Autodesk Fusion 360 part; units mm, degrees
(part 2 of 10)
  line L884 (3.8217, -13.8798) -> (4.0299, -13.8798)
  line L885 (4.0299, -13.8798) -> (4.0984, -13.8456)
  line L886 (4.0984, -13.8456) -> (4.1288, -13.8152)
  line L887 (4.1288, -13.8152) -> (4.1631, -13.7466)
  line L888 (4.1631, -13.7466) -> (4.1631, -13.6868)
  line L889 (4.1631, -13.6868) -> (4.1288, -13.6183)
  line L890 (4.1288, -13.6183) -> (4.0984, -13.5879)
  line L891 (4.0984, -13.5879) -> (4.0214, -13.5494)
  line L892 (4.0214, -13.5494) -> (3.839, -13.5038)
  line L893 (3.839, -13.5038) -> (3.8379, -13.5034)
  line L894 (3.8379, -13.5034) -> (3.8373, -13.5033)
  line L895 (3.8373, -13.5033) -> (3.8312, -13.501)
  line L896 (3.8312, -13.501) -> (3.8251, -13.4988)
  line L897 (3.8251, -13.4988) -> (3.8247, -13.4985)
  line L898 (3.8247, -13.4985) -> (3.8236, -13.4981)
  line L899 (3.8236, -13.4981) -> (3.7284, -13.4505)
  line L900 (3.7284, -13.4505) -> (3.7221, -13.4465)
  line L901 (3.7221, -13.4465) -> (3.7202, -13.4458)
  line L902 (3.7202, -13.4458) -> (3.7182, -13.4441)
  line L903 (3.7182, -13.4441) -> (3.7159, -13.4426)
  line L904 (3.7159, -13.4426) -> (3.7146, -13.4411)
  line L905 (3.7146, -13.4411) -> (3.7089, -13.4364)
  line L906 (3.7089, -13.4364) -> (3.6613, -13.3888)
  line L907 (3.6613, -13.3888) -> (3.6565, -13.3831)
  line L908 (3.6565, -13.3831) -> (3.655, -13.3818)
  line L909 (3.655, -13.3818) -> (3.6536, -13.3795)
  line L910 (3.6536, -13.3795) -> (3.6519, -13.3774)
  line L911 (3.6519, -13.3774) -> (3.6512, -13.3756)
  line L912 (3.6512, -13.3756) -> (3.6472, -13.3693)
  line L913 (3.6472, -13.3693) -> (3.5996, -13.2741)
  line L914 (3.5996, -13.2741) -> (3.5943, -13.2603)
  line L915 (3.5943, -13.2603) -> (3.5941, -13.2577)
  line L916 (3.5941, -13.2577) -> (3.5931, -13.2552)
  line L917 (3.5931, -13.2552) -> (3.5917, -13.2405)
  line L918 (3.5917, -13.2405) -> (3.5917, -13.1453)
  line L919 (3.5917, -13.1453) -> (3.5931, -13.1307)
  line L920 (3.5931, -13.1307) -> (3.5941, -13.1282)
  line L921 (3.5941, -13.1282) -> (3.5943, -13.1255)
  line L922 (3.5943, -13.1255) -> (3.5996, -13.1118)
  line L923 (3.5996, -13.1118) -> (3.6472, -13.0165)
  line L924 (3.6472, -13.0165) -> (3.6512, -13.0102)
  line L925 (3.6512, -13.0102) -> (3.6519, -13.0084)
  line L926 (3.6519, -13.0084) -> (3.6536, -13.0063)
  line L927 (3.6536, -13.0063) -> (3.655, -13.0041)
  line L928 (3.655, -13.0041) -> (3.6565, -13.0028)
  line L929 (3.6565, -13.0028) -> (3.6613, -12.997)
  line L930 (3.6613, -12.997) -> (3.7089, -12.9494)
  line L931 (3.7089, -12.9494) -> (3.7146, -12.9447)
  line L932 (3.7146, -12.9447) -> (3.7159, -12.9432)
  line L933 (3.7159, -12.9432) -> (3.7182, -12.9418)
  line L934 (3.7182, -12.9418) -> (3.7202, -12.9401)
  line L935 (3.7202, -12.9401) -> (3.7221, -12.9393)
  line L936 (3.7221, -12.9393) -> (3.7284, -12.9354)
  line L937 (3.7284, -12.9354) -> (3.8236, -12.8877)
  line L938 (3.8236, -12.8877) -> (3.8373, -12.8825)
  line L939 (3.8373, -12.8825) -> (3.84, -12.8823)
  line L940 (3.84, -12.8823) -> (3.8425, -12.8813)
  line L941 (3.8425, -12.8813) -> (3.8571, -12.8798)
  line L942 (3.8571, -12.8798) -> (4.0952, -12.8798)
  line L943 (4.0952, -12.8798) -> (4.1026, -12.8805)
  line L944 (5.4598, -12.8867) -> (5.4836, -12.9038)
  line L945 (5.4836, -12.9038) -> (5.4989, -12.9287)
  line L946 (5.4989, -12.9287) -> (5.5035, -12.9576)
  line L947 (5.5035, -12.9576) -> (5.5015, -12.9722)
  line L948 (5.5015, -12.9722) -> (5.2634, -13.9722)
  line L949 (5.2634, -13.9722) -> (5.2617, -13.9772)
  line L950 (5.2617, -13.9772) -> (5.2615, -13.979)
  line L951 (5.2615, -13.979) -> (5.2605, -13.9806)
  line L952 (5.2605, -13.9806) -> (5.2586, -13.9861)
  line L953 (5.2586, -13.9861) -> (5.2523, -13.9949)
  line L954 (5.2523, -13.9949) -> (5.2468, -14.0043)
  line L955 (5.2468, -14.0043) -> (5.2437, -14.0067)
  line L956 (5.2437, -14.0067) -> (5.2415, -14.0098)
  line L957 (5.2415, -14.0098) -> (5.2322, -14.0155)
  line L958 (5.2322, -14.0155) -> (5.2236, -14.0221)
  line L959 (5.2236, -14.0221) -> (5.2198, -14.0231)
  line L960 (5.2198, -14.0231) -> (5.2166, -14.0251)
  line L961 (5.2166, -14.0251) -> (5.2058, -14.0269)
  line L962 (5.2058, -14.0269) -> (5.1953, -14.0297)
  line L963 (5.1953, -14.0297) -> (5.1915, -14.0292)
  line L964 (5.1915, -14.0292) -> (5.1877, -14.0298)
  line L965 (5.1877, -14.0298) -> (5.1771, -14.0272)
  line L966 (5.1771, -14.0272) -> (5.1663, -14.0258)
  line L967 (5.1663, -14.0258) -> (5.163, -14.0239)
  line L968 (5.163, -14.0239) -> (5.1592, -14.023)
  line L969 (5.1592, -14.023) -> (5.1504, -14.0166)
  line L970 (5.1504, -14.0166) -> (5.141, -14.0111)
  line L971 (5.141, -14.0111) -> (5.1386, -14.0081)
  line L972 (5.1386, -14.0081) -> (5.1355, -14.0058)
  line L973 (5.1355, -14.0058) -> (5.1298, -13.9966)
  line L974 (5.1298, -13.9966) -> (5.1232, -13.9879)
  line L975 (5.1232, -13.9879) -> (5.1211, -13.9825)
  line L976 (5.1211, -13.9825) -> (5.1202, -13.9809)
  line L977 (5.1202, -13.9809) -> (5.1199, -13.9791)
  line L978 (5.1199, -13.9791) -> (5.118, -13.9741)
  line L979 (5.118, -13.9741) -> (5, -13.5316)
  line L980 (5, -13.5316) -> (4.882, -13.9741)
  line L981 (4.882, -13.9741) -> (4.8801, -13.9791)
  line L982 (4.8801, -13.9791) -> (4.8798, -13.9809)
  line L983 (4.8798, -13.9809) -> (4.8789, -13.9825)
  line L984 (4.8789, -13.9825) -> (4.8768, -13.9879)
  line L985 (4.8768, -13.9879) -> (4.8702, -13.9966)
  line L986 (4.8702, -13.9966) -> (4.8645, -14.0058)
  line L987 (4.8645, -14.0058) -> (4.8614, -14.0081)
  line L988 (4.8614, -14.0081) -> (4.859, -14.0111)
  line L989 (4.859, -14.0111) -> (4.8496, -14.0166)
  line L990 (4.8496, -14.0166) -> (4.8408, -14.023)
  line L991 (4.8408, -14.023) -> (4.837, -14.0239)
  line L992 (4.837, -14.0239) -> (4.8337, -14.0258)
  line L993 (4.8337, -14.0258) -> (4.8229, -14.0272)
  line L994 (4.8229, -14.0272) -> (4.8123, -14.0298)
  line L995 (4.8123, -14.0298) -> (4.8085, -14.0292)
  line L996 (4.8085, -14.0292) -> (4.8047, -14.0297)
  line L997 (4.8047, -14.0297) -> (4.7942, -14.0269)
  line L998 (4.7942, -14.0269) -> (4.7834, -14.0251)
  line L999 (4.7834, -14.0251) -> (4.7802, -14.0231)
  line L1000 (4.7802, -14.0231) -> (4.7764, -14.0221)
  line L1001 (4.7764, -14.0221) -> (4.7678, -14.0155)
  line L1002 (4.7678, -14.0155) -> (4.7585, -14.0098)
  line L1003 (4.7585, -14.0098) -> (4.7563, -14.0067)
  line L1004 (4.7563, -14.0067) -> (4.7532, -14.0043)
  line L1005 (4.7532, -14.0043) -> (4.7477, -13.9949)
  line L1006 (4.7477, -13.9949) -> (4.7414, -13.9861)
  line L1007 (4.7414, -13.9861) -> (4.7395, -13.9806)
  line L1008 (4.7395, -13.9806) -> (4.7385, -13.979)
  line L1009 (4.7385, -13.979) -> (4.7383, -13.9772)
  line L1010 (4.7383, -13.9772) -> (4.7366, -13.9722)
  line L1011 (4.7366, -13.9722) -> (4.4985, -12.9722)
  line L1012 (4.4985, -12.9722) -> (4.4965, -12.9576)
  line L1013 (4.4965, -12.9576) -> (4.5011, -12.9287)
  line L1014 (4.5011, -12.9287) -> (4.5164, -12.9038)
  line L1015 (4.5164, -12.9038) -> (4.5402, -12.8866)
  line L1016 (4.5402, -12.8866) -> (4.5686, -12.8799)
  line L1017 (4.5686, -12.8799) -> (4.5975, -12.8845)
  line L1018 (4.5975, -12.8845) -> (4.6224, -12.8998)
  line L1019 (4.6224, -12.8998) -> (4.6396, -12.9235)
  line L1020 (4.6396, -12.9235) -> (4.6444, -12.9374)
  line L1021 (4.6444, -12.9374) -> (4.8136, -13.6483)
  line L1022 (4.8136, -13.6483) -> (4.9275, -13.2212)
  line L1023 (4.9275, -13.2212) -> (4.9288, -13.2178)
  line L1024 (4.9288, -13.2178) -> (4.929, -13.2163)
  line L1025 (4.929, -13.2163) -> (4.93, -13.2146)
  line L1026 (4.93, -13.2146) -> (4.9327, -13.2074)
  line L1027 (4.9327, -13.2074) -> (4.9387, -13.1996)
  line L1028 (4.9387, -13.1996) -> (4.9437, -13.191)
  line L1029 (4.9437, -13.191) -> (4.9475, -13.1881)
  line L1030 (4.9475, -13.1881) -> (4.9505, -13.1842)
  line L1031 (4.9505, -13.1842) -> (4.959, -13.1792)
  line L1032 (4.959, -13.1792) -> (4.9669, -13.1732)
  line L1033 (4.9669, -13.1732) -> (4.9716, -13.172)
  line L1034 (4.9716, -13.172) -> (4.9758, -13.1695)
  line L1035 (4.9758, -13.1695) -> (4.9856, -13.1682)
  line L1036 (4.9856, -13.1682) -> (4.9952, -13.1657)
  line L1037 (4.9952, -13.1657) -> (5, -13.1663)
  line L1038 (5, -13.1663) -> (5.0048, -13.1657)
  line L1039 (5.0048, -13.1657) -> (5.0144, -13.1682)
  line L1040 (5.0144, -13.1682) -> (5.0242, -13.1695)
  line L1041 (5.0242, -13.1695) -> (5.0284, -13.172)
  line L1042 (5.0284, -13.172) -> (5.0331, -13.1732)
  line L1043 (5.0331, -13.1732) -> (5.041, -13.1792)
  line L1044 (5.041, -13.1792) -> (5.0495, -13.1842)
  line L1045 (5.0495, -13.1842) -> (5.0525, -13.1881)
  line L1046 (5.0525, -13.1881) -> (5.0563, -13.191)
  line L1047 (5.0563, -13.191) -> (5.0613, -13.1996)
  line L1048 (5.0613, -13.1996) -> (5.0673, -13.2074)
  line L1049 (5.0673, -13.2074) -> (5.07, -13.2146)
  line L1050 (5.07, -13.2146) -> (5.071, -13.2163)
  line L1051 (5.071, -13.2163) -> (5.0712, -13.2178)
  line L1052 (5.0712, -13.2178) -> (5.0725, -13.2212)
  line L1053 (5.0725, -13.2212) -> (5.1864, -13.6483)
  line L1054 (5.1864, -13.6483) -> (5.3556, -12.9374)
  line L1055 (5.3556, -12.9374) -> (5.3604, -12.9235)
  line L1056 (5.3604, -12.9235) -> (5.3776, -12.8998)
  line L1057 (5.3776, -12.8998) -> (5.4025, -12.8845)
  line L1058 (5.4025, -12.8845) -> (5.4314, -12.8799)
  line L1059 (5.4314, -12.8799) -> (5.4598, -12.8867)
  line L1060 (6.0371, -12.842) -> (6.0592, -12.8612)
  line L1061 (6.0592, -12.8612) -> (6.0723, -12.8874)
  line L1062 (6.0723, -12.8874) -> (6.0744, -12.9166)
  line L1063 (6.0744, -12.9166) -> (6.0712, -12.9309)
  line L1064 (6.0712, -12.9309) -> (5.866, -13.5465)
  line L1065 (5.866, -13.5465) -> (6.1631, -13.5465)
  line L1066 (6.1631, -13.5465) -> (6.1631, -13.2882)
  line L1067 (6.1631, -13.2882) -> (6.1645, -13.2735)
  line L1068 (6.1645, -13.2735) -> (6.1757, -13.2465)
  line L1069 (6.1757, -13.2465) -> (6.1964, -13.2258)
  line L1070 (6.1964, -13.2258) -> (6.2235, -13.2146)
  line L1071 (6.2235, -13.2146) -> (6.2527, -13.2146)
  line L1072 (6.2527, -13.2146) -> (6.2798, -13.2258)
  line L1073 (6.2798, -13.2258) -> (6.3005, -13.2465)
  line L1074 (6.3005, -13.2465) -> (6.3117, -13.2735)
  line L1075 (6.3117, -13.2735) -> (6.3131, -13.2882)
  line L1076 (6.3131, -13.2882) -> (6.3131, -13.5465)
  line L1077 (6.3131, -13.5465) -> (6.381, -13.5465)
  line L1078 (6.381, -13.5465) -> (6.3956, -13.5479)
  line L1079 (6.3956, -13.5479) -> (6.4226, -13.5591)
  line L1080 (6.4226, -13.5591) -> (6.4433, -13.5798)
  line L1081 (6.4433, -13.5798) -> (6.4545, -13.6069)
  line L1082 (6.4545, -13.6069) -> (6.4545, -13.6361)
  line L1083 (6.4545, -13.6361) -> (6.4433, -13.6632)
  line L1084 (6.4433, -13.6632) -> (6.4226, -13.6838)
  line L1085 (6.4226, -13.6838) -> (6.3956, -13.695)
  line L1086 (6.3956, -13.695) -> (6.381, -13.6965)
  line L1087 (6.381, -13.6965) -> (6.3131, -13.6965)
  line L1088 (6.3131, -13.6965) -> (6.3131, -13.9548)
  line L1089 (6.3131, -13.9548) -> (6.3117, -13.9695)
  line L1090 (6.3117, -13.9695) -> (6.3005, -13.9965)
  line L1091 (6.3005, -13.9965) -> (6.2798, -14.0172)
  line L1092 (6.2798, -14.0172) -> (6.2527, -14.0284)
  line L1093 (6.2527, -14.0284) -> (6.2235, -14.0284)
  line L1094 (6.2235, -14.0284) -> (6.1964, -14.0172)
  line L1095 (6.1964, -14.0172) -> (6.1757, -13.9965)
  line L1096 (6.1757, -13.9965) -> (6.1645, -13.9695)
  line L1097 (6.1645, -13.9695) -> (6.1631, -13.9548)
  line L1098 (6.1631, -13.9548) -> (6.1631, -13.6965)
  line L1099 (6.1631, -13.6965) -> (5.7619, -13.6965)
  line L1100 (5.7619, -13.6965) -> (5.7545, -13.6958)
  line L1101 (5.7545, -13.6958) -> (5.7525, -13.6959)
  line L1102 (5.7525, -13.6959) -> (5.7511, -13.6954)
  line L1103 (5.7511, -13.6954) -> (5.7473, -13.695)
  line L1104 (5.7473, -13.695) -> (5.7362, -13.6904)
  line L1105 (5.7362, -13.6904) -> (5.7248, -13.6866)
  line L1106 (5.7248, -13.6866) -> (5.7227, -13.6849)
  line L1107 (5.7227, -13.6849) -> (5.7202, -13.6838)
  line L1108 (5.7202, -13.6838) -> (5.7117, -13.6753)
  line L1109 (5.7117, -13.6753) -> (5.7027, -13.6675)
  line L1110 (5.7027, -13.6675) -> (5.7015, -13.6651)
  line L1111 (5.7015, -13.6651) -> (5.6995, -13.6632)
  line L1112 (5.6995, -13.6632) -> (5.6949, -13.652)
  line L1113 (5.6949, -13.652) -> (5.6896, -13.6413)
  line L1114 (5.6896, -13.6413) -> (5.6894, -13.6386)
  line L1115 (5.6894, -13.6386) -> (5.6883, -13.6361)
  line L1116 (5.6883, -13.6361) -> (5.6883, -13.6241)
  line L1117 (5.6883, -13.6241) -> (5.6875, -13.6121)
  line L1118 (5.6875, -13.6121) -> (5.6883, -13.6084)
  line L1119 (5.6883, -13.6084) -> (5.6883, -13.6069)
  line L1120 (5.6883, -13.6069) -> (5.6891, -13.605)
  line L1121 (5.6891, -13.605) -> (5.6908, -13.5978)
  line L1122 (5.6908, -13.5978) -> (5.9288, -12.8835)
  line L1123 (5.9288, -12.8835) -> (5.9348, -12.8701)
  line L1124 (5.9348, -12.8701) -> (5.954, -12.848)
  line L1125 (5.954, -12.848) -> (5.9802, -12.8349)
  line L1126 (5.9802, -12.8349) -> (6.0094, -12.8328)
  line L1127 (6.0094, -12.8328) -> (6.0371, -12.842)
  line L1128 (14.338, -11.4596) -> (14.3704, -11.492)
  line L1129 (14.3704, -11.492) -> (14.375, -11.515)
  line L1130 (14.375, -11.515) -> (14.375, -25.485)
  line L1131 (14.375, -25.485) -> (14.3704, -25.508)
  line L1132 (14.3704, -25.508) -> (14.338, -25.5404)
  line L1133 (14.338, -25.5404) -> (14.315, -25.545)
  line L1134 (14.315, -25.545) -> (0.345, -25.545)
  line L1135 (0.345, -25.545) -> (0.322, -25.5404)
  line L1136 (0.322, -25.5404) -> (0.2896, -25.508)
  line L1137 (0.2896, -25.508) -> (0.285, -25.485)
  line L1138 (0.285, -25.485) -> (0.285, -11.515)
  line L1139 (0.285, -11.515) -> (0.2896, -11.492)
  line L1140 (0.2896, -11.492) -> (0.322, -11.4596)
  line L1141 (0.322, -11.4596) -> (0.345, -11.455)
  line L1142 (0.345, -11.455) -> (14.315, -11.455)
  line L1143 (14.315, -11.455) -> (14.338, -11.4596)
  line L1144 (0.405, -11.575) -> (0.405, -25.425)
  line L1145 (0.405, -25.425) -> (14.255, -25.425)
  line L1146 (14.255, -25.425) -> (14.255, -11.575)
  line L1147 (14.255, -11.575) -> (0.405, -11.575)
  line L1148 (19.1026, -12.8805) -> (19.1046, -12.8804)
  line L1149 (19.1046, -12.8804) -> (19.1072, -12.881)
  line L1150 (19.1072, -12.881) -> (19.1099, -12.8813)
  line L1151 (19.1099, -12.8813) -> (19.1117, -12.882)
  line L1152 (19.1117, -12.882) -> (19.119, -12.8837)
  line L1153 (19.119, -12.8837) -> (19.2618, -12.9313)
  line L1154 (19.2618, -12.9313) -> (19.2752, -12.9373)
  line L1155 (19.2752, -12.9373) -> (19.2973, -12.9565)
  line L1156 (19.2973, -12.9565) -> (19.3104, -12.9826)
  line L1157 (19.3104, -12.9826) -> (19.3125, -13.0118)
  line L1158 (19.3125, -13.0118) -> (19.3033, -13.0396)
  line L1159 (19.3033, -13.0396) -> (19.2841, -13.0617)
  line L1160 (19.2841, -13.0617) -> (19.2579, -13.0748)
  line L1161 (19.2579, -13.0748) -> (19.2287, -13.0768)
  line L1162 (19.2287, -13.0768) -> (19.2144, -13.0736)
  line L1163 (19.2144, -13.0736) -> (19.0831, -13.0298)
  line L1164 (19.0831, -13.0298) -> (18.8748, -13.0298)
  line L1165 (18.8748, -13.0298) -> (18.8063, -13.0641)
  line L1166 (18.8063, -13.0641) -> (18.7759, -13.0945)
  line L1167 (18.7759, -13.0945) -> (18.7417, -13.163)
  line L1168 (18.7417, -13.163) -> (18.7417, -13.2228)
  line L1169 (18.7417, -13.2228) -> (18.7759, -13.2913)
  line L1170 (18.7759, -13.2913) -> (18.8063, -13.3218)
  line L1171 (18.8063, -13.3218) -> (18.8833, -13.3602)
  line L1172 (18.8833, -13.3602) -> (19.0658, -13.4059)
  line L1173 (19.0658, -13.4059) -> (19.0669, -13.4063)
  line L1174 (19.0669, -13.4063) -> (19.0674, -13.4063)
  line L1175 (19.0674, -13.4063) -> (19.0735, -13.4086)
  line L1176 (19.0735, -13.4086) -> (19.0797, -13.4108)
  line L1177 (19.0797, -13.4108) -> (19.0801, -13.4111)
  line L1178 (19.0801, -13.4111) -> (19.0812, -13.4115)
  line L1179 (19.0812, -13.4115) -> (19.1764, -13.4592)
  line L1180 (19.1764, -13.4592) -> (19.1827, -13.4631)
  line L1181 (19.1827, -13.4631) -> (19.1845, -13.4639)
  line L1182 (19.1845, -13.4639) -> (19.1866, -13.4656)
  line L1183 (19.1866, -13.4656) -> (19.1888, -13.467)
  line L1184 (19.1888, -13.467) -> (19.1901, -13.4685)
  line L1185 (19.1901, -13.4685) -> (19.1959, -13.4732)
  line L1186 (19.1959, -13.4732) -> (19.2435, -13.5208)
  line L1187 (19.2435, -13.5208) -> (19.2482, -13.5266)
  line L1188 (19.2482, -13.5266) -> (19.2497, -13.5279)
  line L1189 (19.2497, -13.5279) -> (19.2511, -13.5301)
  line L1190 (19.2511, -13.5301) -> (19.2528, -13.5322)
  line L1191 (19.2528, -13.5322) -> (19.2536, -13.534)
  line L1192 (19.2536, -13.534) -> (19.2576, -13.5403)
  line L1193 (19.2576, -13.5403) -> (19.3052, -13.6356)
  line L1194 (19.3052, -13.6356) -> (19.3104, -13.6493)
  line L1195 (19.3104, -13.6493) -> (19.3106, -13.652)
  line L1196 (19.3106, -13.652) -> (19.3117, -13.6545)
  line L1197 (19.3117, -13.6545) -> (19.3131, -13.6691)
  line L1198 (19.3131, -13.6691) -> (19.3131, -13.7643)
  line L1199 (19.3131, -13.7643) -> (19.3117, -13.779)
  line L1200 (19.3117, -13.779) -> (19.3106, -13.7815)
  line L1201 (19.3106, -13.7815) -> (19.3104, -13.7842)
  line L1202 (19.3104, -13.7842) -> (19.3052, -13.7979)
  line L1203 (19.3052, -13.7979) -> (19.2576, -13.8931)
  line L1204 (19.2576, -13.8931) -> (19.2536, -13.8994)
  line L1205 (19.2536, -13.8994) -> (19.2528, -13.9012)
  line L1206 (19.2528, -13.9012) -> (19.2511, -13.9033)
  line L1207 (19.2511, -13.9033) -> (19.2497, -13.9056)
  line L1208 (19.2497, -13.9056) -> (19.2482, -13.9069)
  line L1209 (19.2482, -13.9069) -> (19.2435, -13.9126)
  line L1210 (19.2435, -13.9126) -> (19.1959, -13.9602)
  line L1211 (19.1959, -13.9602) -> (19.1901, -13.9649)
  line L1212 (19.1901, -13.9649) -> (19.1888, -13.9664)
  line L1213 (19.1888, -13.9664) -> (19.1866, -13.9679)
  line L1214 (19.1866, -13.9679) -> (19.1845, -13.9696)
  line L1215 (19.1845, -13.9696) -> (19.1827, -13.9703)
  line L1216 (19.1827, -13.9703) -> (19.1764, -13.9743)
  line L1217 (19.1764, -13.9743) -> (19.0812, -14.0219)
  line L1218 (19.0812, -14.0219) -> (19.0674, -14.0272)
  line L1219 (19.0674, -14.0272) -> (19.0647, -14.0273)
  line L1220 (19.0647, -14.0273) -> (19.0623, -14.0284)
  line L1221 (19.0623, -14.0284) -> (19.0476, -14.0298)
  line L1222 (19.0476, -14.0298) -> (18.8095, -14.0298)
  line L1223 (18.8095, -14.0298) -> (18.8021, -14.0291)
  line L1224 (18.8021, -14.0291) -> (18.8001, -14.0292)
  line L1225 (18.8001, -14.0292) -> (18.7975, -14.0286)
  line L1226 (18.7975, -14.0286) -> (18.7949, -14.0284)
  line L1227 (18.7949, -14.0284) -> (18.7931, -14.0276)
  line L1228 (18.7931, -14.0276) -> (18.7858, -14.026)
  line L1229 (18.7858, -14.026) -> (18.6429, -13.9784)
  line L1230 (18.6429, -13.9784) -> (18.6295, -13.9724)
  line L1231 (18.6295, -13.9724) -> (18.6074, -13.9532)
  line L1232 (18.6074, -13.9532) -> (18.5943, -13.927)
  line L1233 (18.5943, -13.927) -> (18.5923, -13.8978)
  line L1234 (18.5923, -13.8978) -> (18.6015, -13.8701)
  line L1235 (18.6015, -13.8701) -> (18.6207, -13.848)
  line L1236 (18.6207, -13.848) -> (18.6469, -13.8349)
  line L1237 (18.6469, -13.8349) -> (18.676, -13.8328)
  line L1238 (18.676, -13.8328) -> (18.6904, -13.836)
  line L1239 (18.6904, -13.836) -> (18.8217, -13.8798)
  line L1240 (18.8217, -13.8798) -> (19.0299, -13.8798)
  line L1241 (19.0299, -13.8798) -> (19.0984, -13.8456)
  line L1242 (19.0984, -13.8456) -> (19.1288, -13.8152)
  line L1243 (19.1288, -13.8152) -> (19.1631, -13.7466)
  line L1244 (19.1631, -13.7466) -> (19.1631, -13.6868)
  line L1245 (19.1631, -13.6868) -> (19.1288, -13.6183)
  line L1246 (19.1288, -13.6183) -> (19.0984, -13.5879)
  line L1247 (19.0984, -13.5879) -> (19.0214, -13.5494)
  line L1248 (19.0214, -13.5494) -> (18.839, -13.5038)
  line L1249 (18.839, -13.5038) -> (18.8379, -13.5034)
  line L1250 (18.8379, -13.5034) -> (18.8373, -13.5033)
  line L1251 (18.8373, -13.5033) -> (18.8312, -13.501)
  line L1252 (18.8312, -13.501) -> (18.8251, -13.4988)
  line L1253 (18.8251, -13.4988) -> (18.8247, -13.4985)
  line L1254 (18.8247, -13.4985) -> (18.8236, -13.4981)
  line L1255 (18.8236, -13.4981) -> (18.7284, -13.4505)
  line L1256 (18.7284, -13.4505) -> (18.7221, -13.4465)
  line L1257 (18.7221, -13.4465) -> (18.7202, -13.4458)
  line L1258 (18.7202, -13.4458) -> (18.7182, -13.4441)
  line L1259 (18.7182, -13.4441) -> (18.7159, -13.4426)
  line L1260 (18.7159, -13.4426) -> (18.7146, -13.4411)
  line L1261 (18.7146, -13.4411) -> (18.7089, -13.4364)
  line L1262 (18.7089, -13.4364) -> (18.6613, -13.3888)
  line L1263 (18.6613, -13.3888) -> (18.6565, -13.3831)
  line L1264 (18.6565, -13.3831) -> (18.655, -13.3818)
  line L1265 (18.655, -13.3818) -> (18.6536, -13.3795)
  line L1266 (18.6536, -13.3795) -> (18.6519, -13.3774)
  line L1267 (18.6519, -13.3774) -> (18.6512, -13.3756)
  line L1268 (18.6512, -13.3756) -> (18.6472, -13.3693)
  line L1269 (18.6472, -13.3693) -> (18.5996, -13.2741)
  line L1270 (18.5996, -13.2741) -> (18.5943, -13.2603)
  line L1271 (18.5943, -13.2603) -> (18.5941, -13.2577)
  line L1272 (18.5941, -13.2577) -> (18.5931, -13.2552)
  line L1273 (18.5931, -13.2552) -> (18.5917, -13.2405)
  line L1274 (18.5917, -13.2405) -> (18.5917, -13.1453)
  line L1275 (18.5917, -13.1453) -> (18.5931, -13.1307)
  line L1276 (18.5931, -13.1307) -> (18.5941, -13.1282)
  line L1277 (18.5941, -13.1282) -> (18.5943, -13.1255)
  line L1278 (18.5943, -13.1255) -> (18.5996, -13.1118)
  line L1279 (18.5996, -13.1118) -> (18.6472, -13.0165)
  line L1280 (18.6472, -13.0165) -> (18.6512, -13.0102)
  line L1281 (18.6512, -13.0102) -> (18.6519, -13.0084)
  line L1282 (18.6519, -13.0084) -> (18.6536, -13.0063)
  line L1283 (18.6536, -13.0063) -> (18.655, -13.0041)
  line L1284 (18.655, -13.0041) -> (18.6565, -13.0028)
  line L1285 (18.6565, -13.0028) -> (18.6613, -12.997)
  line L1286 (18.6613, -12.997) -> (18.7089, -12.9494)
  line L1287 (18.7089, -12.9494) -> (18.7146, -12.9447)
  line L1288 (18.7146, -12.9447) -> (18.7159, -12.9432)
  line L1289 (18.7159, -12.9432) -> (18.7182, -12.9418)
  line L1290 (18.7182, -12.9418) -> (18.7202, -12.9401)
  line L1291 (18.7202, -12.9401) -> (18.7221, -12.9393)
  line L1292 (18.7221, -12.9393) -> (18.7284, -12.9354)
  line L1293 (18.7284, -12.9354) -> (18.8236, -12.8877)
  line L1294 (18.8236, -12.8877) -> (18.8373, -12.8825)
  line L1295 (18.8373, -12.8825) -> (18.84, -12.8823)
  line L1296 (18.84, -12.8823) -> (18.8425, -12.8813)
  line L1297 (18.8425, -12.8813) -> (18.8571, -12.8798)
  line L1298 (18.8571, -12.8798) -> (19.0952, -12.8798)
  line L1299 (19.0952, -12.8798) -> (19.1026, -12.8805)
  line L1300 (20.4598, -12.8867) -> (20.4836, -12.9038)
  line L1301 (20.4836, -12.9038) -> (20.4989, -12.9287)
  line L1302 (20.4989, -12.9287) -> (20.5035, -12.9576)
  line L1303 (20.5035, -12.9576) -> (20.5015, -12.9722)
  line L1304 (20.5015, -12.9722) -> (20.2634, -13.9722)
  line L1305 (20.2634, -13.9722) -> (20.2617, -13.9772)
  line L1306 (20.2617, -13.9772) -> (20.2615, -13.979)
  line L1307 (20.2615, -13.979) -> (20.2605, -13.9806)
  line L1308 (20.2605, -13.9806) -> (20.2586, -13.9861)
  line L1309 (20.2586, -13.9861) -> (20.2523, -13.9949)
  line L1310 (20.2523, -13.9949) -> (20.2468, -14.0043)
  line L1311 (20.2468, -14.0043) -> (20.2437, -14.0067)
  line L1312 (20.2437, -14.0067) -> (20.2415, -14.0098)
  line L1313 (20.2415, -14.0098) -> (20.2322, -14.0155)
  line L1314 (20.2322, -14.0155) -> (20.2236, -14.0221)
  line L1315 (20.2236, -14.0221) -> (20.2198, -14.0231)
  line L1316 (20.2198, -14.0231) -> (20.2166, -14.0251)
  line L1317 (20.2166, -14.0251) -> (20.2058, -14.0269)
  line L1318 (20.2058, -14.0269) -> (20.1953, -14.0297)
  line L1319 (20.1953, -14.0297) -> (20.1915, -14.0292)
  line L1320 (20.1915, -14.0292) -> (20.1877, -14.0298)
  line L1321 (20.1877, -14.0298) -> (20.1771, -14.0272)
  line L1322 (20.1771, -14.0272) -> (20.1663, -14.0258)
  line L1323 (20.1663, -14.0258) -> (20.163, -14.0239)
  line L1324 (20.163, -14.0239) -> (20.1592, -14.023)
  line L1325 (20.1592, -14.023) -> (20.1504, -14.0166)
  line L1326 (20.1504, -14.0166) -> (20.141, -14.0111)
  line L1327 (20.141, -14.0111) -> (20.1386, -14.0081)
  line L1328 (20.1386, -14.0081) -> (20.1355, -14.0058)
  line L1329 (20.1355, -14.0058) -> (20.1298, -13.9966)
  line L1330 (20.1298, -13.9966) -> (20.1232, -13.9879)
  line L1331 (20.1232, -13.9879) -> (20.1211, -13.9825)
  line L1332 (20.1211, -13.9825) -> (20.1202, -13.9809)
  line L1333 (20.1202, -13.9809) -> (20.1199, -13.9791)
  line L1334 (20.1199, -13.9791) -> (20.118, -13.9741)
  line L1335 (20.118, -13.9741) -> (20, -13.5316)
  line L1336 (20, -13.5316) -> (19.882, -13.9741)
  line L1337 (19.882, -13.9741) -> (19.8801, -13.9791)
  line L1338 (19.8801, -13.9791) -> (19.8798, -13.9809)
  line L1339 (19.8798, -13.9809) -> (19.8789, -13.9825)
  line L1340 (19.8789, -13.9825) -> (19.8768, -13.9879)
  line L1341 (19.8768, -13.9879) -> (19.8702, -13.9966)
  line L1342 (19.8702, -13.9966) -> (19.8645, -14.0058)
  line L1343 (19.8645, -14.0058) -> (19.8614, -14.0081)
  line L1344 (19.8614, -14.0081) -> (19.859, -14.0111)
  line L1345 (19.859, -14.0111) -> (19.8496, -14.0166)
  line L1346 (19.8496, -14.0166) -> (19.8408, -14.023)
  line L1347 (19.8408, -14.023) -> (19.837, -14.0239)
  line L1348 (19.837, -14.0239) -> (19.8337, -14.0258)
  line L1349 (19.8337, -14.0258) -> (19.8229, -14.0272)
  line L1350 (19.8229, -14.0272) -> (19.8123, -14.0298)
  line L1351 (19.8123, -14.0298) -> (19.8085, -14.0292)
  line L1352 (19.8085, -14.0292) -> (19.8047, -14.0297)
  line L1353 (19.8047, -14.0297) -> (19.7942, -14.0269)
  line L1354 (19.7942, -14.0269) -> (19.7834, -14.0251)
  line L1355 (19.7834, -14.0251) -> (19.7802, -14.0231)
  line L1356 (19.7802, -14.0231) -> (19.7764, -14.0221)
  line L1357 (19.7764, -14.0221) -> (19.7678, -14.0155)
  line L1358 (19.7678, -14.0155) -> (19.7585, -14.0098)
  line L1359 (19.7585, -14.0098) -> (19.7563, -14.0067)
  line L1360 (19.7563, -14.0067) -> (19.7532, -14.0043)
  line L1361 (19.7532, -14.0043) -> (19.7477, -13.9949)
  line L1362 (19.7477, -13.9949) -> (19.7414, -13.9861)
  line L1363 (19.7414, -13.9861) -> (19.7395, -13.9806)
  line L1364 (19.7395, -13.9806) -> (19.7385, -13.979)
  line L1365 (19.7385, -13.979) -> (19.7383, -13.9772)
  line L1366 (19.7383, -13.9772) -> (19.7366, -13.9722)
  line L1367 (19.7366, -13.9722) -> (19.4985, -12.9722)
  line L1368 (19.4985, -12.9722) -> (19.4965, -12.9576)
  line L1369 (19.4965, -12.9576) -> (19.5011, -12.9287)
  line L1370 (19.5011, -12.9287) -> (19.5164, -12.9038)
  line L1371 (19.5164, -12.9038) -> (19.5402, -12.8866)
  line L1372 (19.5402, -12.8866) -> (19.5686, -12.8799)
  line L1373 (19.5686, -12.8799) -> (19.5975, -12.8845)
  line L1374 (19.5975, -12.8845) -> (19.6224, -12.8998)
  line L1375 (19.6224, -12.8998) -> (19.6396, -12.9235)
  line L1376 (19.6396, -12.9235) -> (19.6444, -12.9374)
  line L1377 (19.6444, -12.9374) -> (19.8136, -13.6483)
  line L1378 (19.8136, -13.6483) -> (19.9275, -13.2212)
  line L1379 (19.9275, -13.2212) -> (19.9288, -13.2178)
  line L1380 (19.9288, -13.2178) -> (19.929, -13.2163)
  line L1381 (19.929, -13.2163) -> (19.93, -13.2146)
  line L1382 (19.93, -13.2146) -> (19.9327, -13.2074)
  line L1383 (19.9327, -13.2074) -> (19.9387, -13.1996)
  line L1384 (19.9387, -13.1996) -> (19.9437, -13.191)
  line L1385 (19.9437, -13.191) -> (19.9475, -13.1881)
  line L1386 (19.9475, -13.1881) -> (19.9505, -13.1842)
  line L1387 (19.9505, -13.1842) -> (19.959, -13.1792)
  line L1388 (19.959, -13.1792) -> (19.9669, -13.1732)
  line L1389 (19.9669, -13.1732) -> (19.9716, -13.172)
  line L1390 (19.9716, -13.172) -> (19.9758, -13.1695)
  line L1391 (19.9758, -13.1695) -> (19.9856, -13.1682)
  line L1392 (19.9856, -13.1682) -> (19.9952, -13.1657)
  line L1393 (19.9952, -13.1657) -> (20, -13.1663)
  line L1394 (20, -13.1663) -> (20.0048, -13.1657)
  line L1395 (20.0048, -13.1657) -> (20.0144, -13.1682)
  line L1396 (20.0144, -13.1682) -> (20.0242, -13.1695)
  line L1397 (20.0242, -13.1695) -> (20.0284, -13.172)
  line L1398 (20.0284, -13.172) -> (20.0331, -13.1732)
  line L1399 (20.0331, -13.1732) -> (20.041, -13.1792)
  line L1400 (20.041, -13.1792) -> (20.0495, -13.1842)
  line L1401 (20.0495, -13.1842) -> (20.0525, -13.1881)
  line L1402 (20.0525, -13.1881) -> (20.0563, -13.191)
  line L1403 (20.0563, -13.191) -> (20.0613, -13.1996)
  line L1404 (20.0613, -13.1996) -> (20.0673, -13.2074)
  line L1405 (20.0673, -13.2074) -> (20.07, -13.2146)
  line L1406 (20.07, -13.2146) -> (20.071, -13.2163)
  line L1407 (20.071, -13.2163) -> (20.0712, -13.2178)
  line L1408 (20.0712, -13.2178) -> (20.0725, -13.2212)
  line L1409 (20.0725, -13.2212) -> (20.1864, -13.6483)
  line L1410 (20.1864, -13.6483) -> (20.3556, -12.9374)
  line L1411 (20.3556, -12.9374) -> (20.3604, -12.9235)
  line L1412 (20.3604, -12.9235) -> (20.3776, -12.8998)
  line L1413 (20.3776, -12.8998) -> (20.4025, -12.8845)
  line L1414 (20.4025, -12.8845) -> (20.4314, -12.8799)
  line L1415 (20.4314, -12.8799) -> (20.4598, -12.8867)
  line L1416 (21.3956, -12.8813) -> (21.396, -12.8814)
  line L1417 (21.396, -12.8814) -> (21.3965, -12.8814)
  line L1418 (21.3965, -12.8814) -> (21.4095, -12.887)
  line L1419 (21.4095, -12.887) -> (21.4226, -12.8925)
  line L1420 (21.4226, -12.8925) -> (21.4229, -12.8928)
  line L1421 (21.4229, -12.8928) -> (21.4234, -12.893)
  line L1422 (21.4234, -12.893) -> (21.4333, -12.9031)
  line L1423 (21.4333, -12.9031) -> (21.4433, -12.9132)
  line L1424 (21.4433, -12.9132) -> (21.4435, -12.9136)
  line L1425 (21.4435, -12.9136) -> (21.4438, -12.9139)
  line L1426 (21.4438, -12.9139) -> (21.4491, -12.9271)
  line L1427 (21.4491, -12.9271) -> (21.4545, -12.9402)
  line L1428 (21.4545, -12.9402) -> (21.4545, -12.9407)
  line L1429 (21.4545, -12.9407) -> (21.4547, -12.9411)
  line L1430 (21.4547, -12.9411) -> (21.4545, -12.9553)
  line L1431 (21.4545, -12.9553) -> (21.4545, -12.9695)
  line L1432 (21.4545, -12.9695) -> (21.4543, -12.9699)
  line L1433 (21.4543, -12.9699) -> (21.4543, -12.9703)
  line L1434 (21.4543, -12.9703) -> (21.4499, -12.9844)
  line L1435 (21.4499, -12.9844) -> (21.0213, -13.9844)
  line L1436 (21.0213, -13.9844) -> (21.0142, -13.9972)
  line L1437 (21.0142, -13.9972) -> (20.9933, -14.0177)
  line L1438 (20.9933, -14.0177) -> (20.9661, -14.0286)
  line L1439 (20.9661, -14.0286) -> (20.9369, -14.0282)
  line L1440 (20.9369, -14.0282) -> (20.91, -14.0167)
  line L1441 (20.91, -14.0167) -> (20.8895, -13.9957)
  line L1442 (20.8895, -13.9957) -> (20.8786, -13.9686)
  line L1443 (20.8786, -13.9686) -> (20.879, -13.9393)
  line L1444 (20.879, -13.9393) -> (20.8834, -13.9253)
  line L1445 (20.8834, -13.9253) -> (21.2672, -13.0298)
  line L1446 (21.2672, -13.0298) -> (20.7143, -13.0298)
  line L1447 (20.7143, -13.0298) -> (20.6997, -13.0284)
  line L1448 (20.6997, -13.0284) -> (20.6726, -13.0172)
  line L1449 (20.6726, -13.0172) -> (20.6519, -12.9965)
  line L1450 (20.6519, -12.9965) -> (20.6407, -12.9695)
  line L1451 (20.6407, -12.9695) -> (20.6407, -12.9402)
  line L1452 (20.6407, -12.9402) -> (20.6519, -12.9132)
  line L1453 (20.6519, -12.9132) -> (20.6726, -12.8925)
  line L1454 (20.6726, -12.8925) -> (20.6997, -12.8813)
  line L1455 (20.6997, -12.8813) -> (20.7143, -12.8798)
  line L1456 (20.7143, -12.8798) -> (21.381, -12.8798)
  line L1457 (21.381, -12.8798) -> (21.3956, -12.8813)
  line L1458 (29.428, -11.4596) -> (29.4604, -11.492)
  line L1459 (29.4604, -11.492) -> (29.465, -11.515)
  line L1460 (29.465, -11.515) -> (29.465, -25.485)
  line L1461 (29.465, -25.485) -> (29.4604, -25.508)
  line L1462 (29.4604, -25.508) -> (29.428, -25.5404)
  line L1463 (29.428, -25.5404) -> (29.405, -25.545)
  line L1464 (29.405, -25.545) -> (15.435, -25.545)
  line L1465 (15.435, -25.545) -> (15.412, -25.5404)
  line L1466 (15.412, -25.5404) -> (15.3796, -25.508)
  line L1467 (15.3796, -25.508) -> (15.375, -25.485)
  line L1468 (15.375, -25.485) -> (15.375, -11.515)
  line L1469 (15.375, -11.515) -> (15.3796, -11.492)
  line L1470 (15.3796, -11.492) -> (15.412, -11.4596)
  line L1471 (15.412, -11.4596) -> (15.435, -11.455)
  line L1472 (15.435, -11.455) -> (29.405, -11.455)
  line L1473 (29.405, -11.455) -> (29.428, -11.4596)
  line L1474 (15.495, -11.575) -> (15.495, -25.425)
  line L1475 (15.495, -25.425) -> (29.345, -25.425)
  line L1476 (29.345, -25.425) -> (29.345, -11.575)
  line L1477 (29.345, -11.575) -> (15.495, -11.575)
  line L1478 (-29.3974, -12.3805) -> (-29.3954, -12.3804)
  line L1479 (-29.3954, -12.3804) -> (-29.3928, -12.381)
  line L1480 (-29.3928, -12.381) -> (-29.3901, -12.3813)
  line L1481 (-29.3901, -12.3813) -> (-29.3883, -12.382)
  line L1482 (-29.3883, -12.382) -> (-29.381, -12.3837)
  line L1483 (-29.381, -12.3837) -> (-29.2382, -12.4313)
  line L1484 (-29.2382, -12.4313) -> (-29.2248, -12.4373)
  line L1485 (-29.2248, -12.4373) -> (-29.2027, -12.4565)
  line L1486 (-29.2027, -12.4565) -> (-29.1896, -12.4826)
  line L1487 (-29.1896, -12.4826) -> (-29.1875, -12.5118)
  line L1488 (-29.1875, -12.5118) -> (-29.1967, -12.5396)
  line L1489 (-29.1967, -12.5396) -> (-29.2159, -12.5617)
  line L1490 (-29.2159, -12.5617) -> (-29.2421, -12.5748)
  line L1491 (-29.2421, -12.5748) -> (-29.2713, -12.5768)
  line L1492 (-29.2713, -12.5768) -> (-29.2856, -12.5736)
  line L1493 (-29.2856, -12.5736) -> (-29.4169, -12.5298)
  line L1494 (-29.4169, -12.5298) -> (-29.6252, -12.5298)
  line L1495 (-29.6252, -12.5298) -> (-29.6937, -12.5641)
  line L1496 (-29.6937, -12.5641) -> (-29.7241, -12.5945)
  line L1497 (-29.7241, -12.5945) -> (-29.7583, -12.663)
  line L1498 (-29.7583, -12.663) -> (-29.7583, -12.7228)
  line L1499 (-29.7583, -12.7228) -> (-29.7241, -12.7913)
  line L1500 (-29.7241, -12.7913) -> (-29.6937, -12.8218)
  line L1501 (-29.6937, -12.8218) -> (-29.6167, -12.8602)
  line L1502 (-29.6167, -12.8602) -> (-29.4342, -12.9059)
  line L1503 (-29.4342, -12.9059) -> (-29.4331, -12.9063)
  line L1504 (-29.4331, -12.9063) -> (-29.4326, -12.9063)
  line L1505 (-29.4326, -12.9063) -> (-29.4265, -12.9086)
  line L1506 (-29.4265, -12.9086) -> (-29.4203, -12.9108)
  line L1507 (-29.4203, -12.9108) -> (-29.4199, -12.9111)
  line L1508 (-29.4199, -12.9111) -> (-29.4188, -12.9115)
  line L1509 (-29.4188, -12.9115) -> (-29.3236, -12.9592)
  line L1510 (-29.3236, -12.9592) -> (-29.3173, -12.9631)
  line L1511 (-29.3173, -12.9631) -> (-29.3155, -12.9639)
  line L1512 (-29.3155, -12.9639) -> (-29.3134, -12.9656)
  line L1513 (-29.3134, -12.9656) -> (-29.3112, -12.967)
  line L1514 (-29.3112, -12.967) -> (-29.3099, -12.9685)
  line L1515 (-29.3099, -12.9685) -> (-29.3041, -12.9732)
  line L1516 (-29.3041, -12.9732) -> (-29.2565, -13.0208)
  line L1517 (-29.2565, -13.0208) -> (-29.2518, -13.0266)
  line L1518 (-29.2518, -13.0266) -> (-29.2503, -13.0279)
  line L1519 (-29.2503, -13.0279) -> (-29.2489, -13.0301)
  line L1520 (-29.2489, -13.0301) -> (-29.2472, -13.0322)
  line L1521 (-29.2472, -13.0322) -> (-29.2464, -13.034)
  line L1522 (-29.2464, -13.034) -> (-29.2424, -13.0403)
  line L1523 (-29.2424, -13.0403) -> (-29.1948, -13.1356)
  line L1524 (-29.1948, -13.1356) -> (-29.1896, -13.1493)
  line L1525 (-29.1896, -13.1493) -> (-29.1894, -13.152)
  line L1526 (-29.1894, -13.152) -> (-29.1883, -13.1545)
  line L1527 (-29.1883, -13.1545) -> (-29.1869, -13.1691)
  line L1528 (-29.1869, -13.1691) -> (-29.1869, -13.2643)
  line L1529 (-29.1869, -13.2643) -> (-29.1883, -13.279)
  line L1530 (-29.1883, -13.279) -> (-29.1894, -13.2815)
  line L1531 (-29.1894, -13.2815) -> (-29.1896, -13.2842)
  line L1532 (-29.1896, -13.2842) -> (-29.1948, -13.2979)
  line L1533 (-29.1948, -13.2979) -> (-29.2424, -13.3931)
  line L1534 (-29.2424, -13.3931) -> (-29.2464, -13.3994)
  line L1535 (-29.2464, -13.3994) -> (-29.2472, -13.4012)
  line L1536 (-29.2472, -13.4012) -> (-29.2489, -13.4033)
  line L1537 (-29.2489, -13.4033) -> (-29.2503, -13.4056)
  line L1538 (-29.2503, -13.4056) -> (-29.2518, -13.4069)
  line L1539 (-29.2518, -13.4069) -> (-29.2565, -13.4126)
  line L1540 (-29.2565, -13.4126) -> (-29.3041, -13.4602)
  line L1541 (-29.3041, -13.4602) -> (-29.3099, -13.4649)
  line L1542 (-29.3099, -13.4649) -> (-29.3112, -13.4665)
  line L1543 (-29.3112, -13.4665) -> (-29.3134, -13.4679)
  line L1544 (-29.3134, -13.4679) -> (-29.3155, -13.4696)
  line L1545 (-29.3155, -13.4696) -> (-29.3173, -13.4703)
  line L1546 (-29.3173, -13.4703) -> (-29.3236, -13.4743)
  line L1547 (-29.3236, -13.4743) -> (-29.4188, -13.5219)
  line L1548 (-29.4188, -13.5219) -> (-29.4326, -13.5272)
  line L1549 (-29.4326, -13.5272) -> (-29.4353, -13.5273)
  line L1550 (-29.4353, -13.5273) -> (-29.4377, -13.5284)
  line L1551 (-29.4377, -13.5284) -> (-29.4524, -13.5298)
  line L1552 (-29.4524, -13.5298) -> (-29.6905, -13.5298)
  line L1553 (-29.6905, -13.5298) -> (-29.6979, -13.5291)
  line L1554 (-29.6979, -13.5291) -> (-29.6999, -13.5292)
  line L1555 (-29.6999, -13.5292) -> (-29.7025, -13.5286)
  line L1556 (-29.7025, -13.5286) -> (-29.7051, -13.5284)
  line L1557 (-29.7051, -13.5284) -> (-29.7069, -13.5276)
  line L1558 (-29.7069, -13.5276) -> (-29.7142, -13.526)
  line L1559 (-29.7142, -13.526) -> (-29.857, -13.4784)
  line L1560 (-29.857, -13.4784) -> (-29.8705, -13.4724)
  line L1561 (-29.8705, -13.4724) -> (-29.8926, -13.4532)
  line L1562 (-29.8926, -13.4532) -> (-29.9057, -13.427)
  line L1563 (-29.9057, -13.427) -> (-29.9077, -13.3978)
  line L1564 (-29.9077, -13.3978) -> (-29.8985, -13.3701)
  line L1565 (-29.8985, -13.3701) -> (-29.8793, -13.3479)
  line L1566 (-29.8793, -13.3479) -> (-29.8531, -13.3349)
  line L1567 (-29.8531, -13.3349) -> (-29.824, -13.3328)
  line L1568 (-29.824, -13.3328) -> (-29.8096, -13.336)
  line L1569 (-29.8096, -13.336) -> (-29.6783, -13.3798)
  line L1570 (-29.6783, -13.3798) -> (-29.4701, -13.3798)
  line L1571 (-29.4701, -13.3798) -> (-29.4016, -13.3456)
  line L1572 (-29.4016, -13.3456) -> (-29.3712, -13.3152)
  line L1573 (-29.3712, -13.3152) -> (-29.3369, -13.2466)
  line L1574 (-29.3369, -13.2466) -> (-29.3369, -13.1868)
  line L1575 (-29.3369, -13.1868) -> (-29.3712, -13.1183)
  line L1576 (-29.3712, -13.1183) -> (-29.4016, -13.0879)
  line L1577 (-29.4016, -13.0879) -> (-29.4786, -13.0494)
  line L1578 (-29.4786, -13.0494) -> (-29.661, -13.0038)
  line L1579 (-29.661, -13.0038) -> (-29.6621, -13.0034)
  line L1580 (-29.6621, -13.0034) -> (-29.6627, -13.0033)
  line L1581 (-29.6627, -13.0033) -> (-29.6688, -13.001)
  line L1582 (-29.6688, -13.001) -> (-29.6749, -12.9988)
  line L1583 (-29.6749, -12.9988) -> (-29.6753, -12.9985)
  line L1584 (-29.6753, -12.9985) -> (-29.6764, -12.9981)
  line L1585 (-29.6764, -12.9981) -> (-29.7716, -12.9505)
  line L1586 (-29.7716, -12.9505) -> (-29.7779, -12.9465)
  line L1587 (-29.7779, -12.9465) -> (-29.7798, -12.9458)
  line L1588 (-29.7798, -12.9458) -> (-29.7818, -12.9441)
  line L1589 (-29.7818, -12.9441) -> (-29.7841, -12.9426)
  line L1590 (-29.7841, -12.9426) -> (-29.7854, -12.9411)
  line L1591 (-29.7854, -12.9411) -> (-29.7911, -12.9364)
  line L1592 (-29.7911, -12.9364) -> (-29.8387, -12.8888)
  line L1593 (-29.8387, -12.8888) -> (-29.8435, -12.8831)
  line L1594 (-29.8435, -12.8831) -> (-29.845, -12.8818)
  line L1595 (-29.845, -12.8818) -> (-29.8464, -12.8795)
  line L1596 (-29.8464, -12.8795) -> (-29.8481, -12.8774)
  line L1597 (-29.8481, -12.8774) -> (-29.8488, -12.8756)
  line L1598 (-29.8488, -12.8756) -> (-29.8528, -12.8693)
  line L1599 (-29.8528, -12.8693) -> (-29.9004, -12.7741)
  line L1600 (-29.9004, -12.7741) -> (-29.9057, -12.7603)
  line L1601 (-29.9057, -12.7603) -> (-29.9059, -12.7577)
  line L1602 (-29.9059, -12.7577) -> (-29.9069, -12.7552)
  line L1603 (-29.9069, -12.7552) -> (-29.9083, -12.7405)
  line L1604 (-29.9083, -12.7405) -> (-29.9083, -12.6453)
  line L1605 (-29.9083, -12.6453) -> (-29.9069, -12.6307)
  line L1606 (-29.9069, -12.6307) -> (-29.9059, -12.6282)
  line L1607 (-29.9059, -12.6282) -> (-29.9057, -12.6255)
  line L1608 (-29.9057, -12.6255) -> (-29.9004, -12.6118)
  line L1609 (-29.9004, -12.6118) -> (-29.8528, -12.5165)
  line L1610 (-29.8528, -12.5165) -> (-29.8488, -12.5102)
  line L1611 (-29.8488, -12.5102) -> (-29.8481, -12.5084)
  line L1612 (-29.8481, -12.5084) -> (-29.8464, -12.5063)
  line L1613 (-29.8464, -12.5063) -> (-29.845, -12.5041)
  line L1614 (-29.845, -12.5041) -> (-29.8435, -12.5028)
  line L1615 (-29.8435, -12.5028) -> (-29.8387, -12.497)
  line L1616 (-29.8387, -12.497) -> (-29.7911, -12.4494)
  line L1617 (-29.7911, -12.4494) -> (-29.7854, -12.4447)
  line L1618 (-29.7854, -12.4447) -> (-29.7841, -12.4432)
  line L1619 (-29.7841, -12.4432) -> (-29.7818, -12.4418)
  line L1620 (-29.7818, -12.4418) -> (-29.7798, -12.4401)
  line L1621 (-29.7798, -12.4401) -> (-29.7779, -12.4393)
  line L1622 (-29.7779, -12.4393) -> (-29.7716, -12.4354)
  line L1623 (-29.7716, -12.4354) -> (-29.6764, -12.3877)
  line L1624 (-29.6764, -12.3877) -> (-29.6627, -12.3825)
  line L1625 (-29.6627, -12.3825) -> (-29.66, -12.3823)
  line L1626 (-29.66, -12.3823) -> (-29.6575, -12.3813)
  line L1627 (-29.6575, -12.3813) -> (-29.6429, -12.3798)
  line L1628 (-29.6429, -12.3798) -> (-29.4048, -12.3798)
  line L1629 (-29.4048, -12.3798) -> (-29.3974, -12.3805)
  line L1630 (-27.3425, -12.3813) -> (-27.34, -12.3823)
  line L1631 (-27.34, -12.3823) -> (-27.3373, -12.3825)
  line L1632 (-27.3373, -12.3825) -> (-27.3236, -12.3877)
  line L1633 (-27.3236, -12.3877) -> (-27.2284, -12.4354)
  line L1634 (-27.2284, -12.4354) -> (-27.2221, -12.4393)
  line L1635 (-27.2221, -12.4393) -> (-27.2202, -12.4401)
  line L1636 (-27.2202, -12.4401) -> (-27.2182, -12.4418)
  line L1637 (-27.2182, -12.4418) -> (-27.2159, -12.4432)
  line L1638 (-27.2159, -12.4432) -> (-27.2146, -12.4447)
  line L1639 (-27.2146, -12.4447) -> (-27.2089, -12.4494)
  line L1640 (-27.2089, -12.4494) -> (-27.1613, -12.497)
  line L1641 (-27.1613, -12.497) -> (-27.1565, -12.5028)
  line L1642 (-27.1565, -12.5028) -> (-27.155, -12.5041)
  line L1643 (-27.155, -12.5041) -> (-27.1536, -12.5063)
  line L1644 (-27.1536, -12.5063) -> (-27.1519, -12.5084)
  line L1645 (-27.1519, -12.5084) -> (-27.1512, -12.5102)
  line L1646 (-27.1512, -12.5102) -> (-27.1472, -12.5165)
  line L1647 (-27.1472, -12.5165) -> (-27.0996, -12.6118)
  line L1648 (-27.0996, -12.6118) -> (-27.0943, -12.6255)
  line L1649 (-27.0943, -12.6255) -> (-27.0941, -12.6282)
  line L1650 (-27.0941, -12.6282) -> (-27.0931, -12.6307)
  line L1651 (-27.0931, -12.6307) -> (-27.0917, -12.6453)
  line L1652 (-27.0917, -12.6453) -> (-27.0917, -12.7405)
  line L1653 (-27.0917, -12.7405) -> (-27.0924, -12.7479)
  line L1654 (-27.0924, -12.7479) -> (-27.0923, -12.7499)
  line L1655 (-27.0923, -12.7499) -> (-27.0928, -12.7525)
  line L1656 (-27.0928, -12.7525) -> (-27.0931, -12.7552)
  line L1657 (-27.0931, -12.7552) -> (-27.0939, -12.757)
  line L1658 (-27.0939, -12.757) -> (-27.0955, -12.7643)
  line L1659 (-27.0955, -12.7643) -> (-27.1431, -12.9071)
  line L1660 (-27.1431, -12.9071) -> (-27.1491, -12.9205)
  line L1661 (-27.1491, -12.9205) -> (-27.1509, -12.9226)
  line L1662 (-27.1509, -12.9226) -> (-27.1519, -12.9251)
  line L1663 (-27.1519, -12.9251) -> (-27.1613, -12.9364)
  line L1664 (-27.1613, -12.9364) -> (-27.6046, -13.3798)
  line L1665 (-27.6046, -13.3798) -> (-27.1667, -13.3798)
  line L1666 (-27.1667, -13.3798) -> (-27.152, -13.3813)
  line L1667 (-27.152, -13.3813) -> (-27.125, -13.3925)
  line L1668 (-27.125, -13.3925) -> (-27.1043, -13.4132)
  line L1669 (-27.1043, -13.4132) -> (-27.0931, -13.4402)
  line L1670 (-27.0931, -13.4402) -> (-27.0931, -13.4695)
  line L1671 (-27.0931, -13.4695) -> (-27.1043, -13.4965)
  line L1672 (-27.1043, -13.4965) -> (-27.125, -13.5172)
  line L1673 (-27.125, -13.5172) -> (-27.152, -13.5284)
  line L1674 (-27.152, -13.5284) -> (-27.1667, -13.5298)
  line L1675 (-27.1667, -13.5298) -> (-27.7857, -13.5298)
  line L1676 (-27.7857, -13.5298) -> (-27.8003, -13.5284)
  line L1677 (-27.8003, -13.5284) -> (-27.8274, -13.5172)
  line L1678 (-27.8274, -13.5172) -> (-27.8481, -13.4965)
  line L1679 (-27.8481, -13.4965) -> (-27.8593, -13.4695)
  line L1680 (-27.8593, -13.4695) -> (-27.8593, -13.4402)
  line L1681 (-27.8593, -13.4402) -> (-27.8481, -13.4132)
  line L1682 (-27.8481, -13.4132) -> (-27.8387, -13.4018)
  line L1683 (-27.8387, -13.4018) -> (-27.2798, -12.8429)
  line L1684 (-27.2798, -12.8429) -> (-27.2417, -12.7284)
  line L1685 (-27.2417, -12.7284) -> (-27.2417, -12.663)
  line L1686 (-27.2417, -12.663) -> (-27.2759, -12.5945)
  line L1687 (-27.2759, -12.5945) -> (-27.3063, -12.5641)
  line L1688 (-27.3063, -12.5641) -> (-27.3748, -12.5298)
  line L1689 (-27.3748, -12.5298) -> (-27.5775, -12.5298)
  line L1690 (-27.5775, -12.5298) -> (-27.646, -12.5641)
  line L1691 (-27.646, -12.5641) -> (-27.6851, -12.6031)
  line L1692 (-27.6851, -12.6031) -> (-27.6964, -12.6124)
  line L1693 (-27.6964, -12.6124) -> (-27.7235, -12.6236)
  line L1694 (-27.7235, -12.6236) -> (-27.7527, -12.6236)
  line L1695 (-27.7527, -12.6236) -> (-27.7798, -12.6124)
  line L1696 (-27.7798, -12.6124) -> (-27.8005, -12.5917)
  line L1697 (-27.8005, -12.5917) -> (-27.8117, -12.5647)
  line L1698 (-27.8117, -12.5647) -> (-27.8117, -12.5354)
  line L1699 (-27.8117, -12.5354) -> (-27.8005, -12.5084)
  line L1700 (-27.8005, -12.5084) -> (-27.7911, -12.497)
  line L1701 (-27.7911, -12.497) -> (-27.7435, -12.4494)
  line L1702 (-27.7435, -12.4494) -> (-27.7378, -12.4447)
  line L1703 (-27.7378, -12.4447) -> (-27.7365, -12.4432)
  line L1704 (-27.7365, -12.4432) -> (-27.7342, -12.4418)
  line L1705 (-27.7342, -12.4418) -> (-27.7321, -12.4401)
  line L1706 (-27.7321, -12.4401) -> (-27.7303, -12.4393)
  line L1707 (-27.7303, -12.4393) -> (-27.724, -12.4354)
  line L1708 (-27.724, -12.4354) -> (-27.6288, -12.3877)
  line L1709 (-27.6288, -12.3877) -> (-27.615, -12.3825)
  line L1710 (-27.615, -12.3825) -> (-27.6124, -12.3823)
  line L1711 (-27.6124, -12.3823) -> (-27.6099, -12.3813)
  line L1712 (-27.6099, -12.3813) -> (-27.5952, -12.3798)
  line L1713 (-27.5952, -12.3798) -> (-27.3571, -12.3798)
  line L1714 (-27.3571, -12.3798) -> (-27.3425, -12.3813)
  line L1715 (-28.0402, -12.3867) -> (-28.0164, -12.4038)
  line L1716 (-28.0164, -12.4038) -> (-28.0011, -12.4287)
  line L1717 (-28.0011, -12.4287) -> (-27.9965, -12.4576)
  line L1718 (-27.9965, -12.4576) -> (-27.9985, -12.4722)
  line L1719 (-27.9985, -12.4722) -> (-28.2366, -13.4722)
  line L1720 (-28.2366, -13.4722) -> (-28.2383, -13.4772)
  line L1721 (-28.2383, -13.4772) -> (-28.2385, -13.479)
  line L1722 (-28.2385, -13.479) -> (-28.2395, -13.4806)
  line L1723 (-28.2395, -13.4806) -> (-28.2414, -13.4861)
  line L1724 (-28.2414, -13.4861) -> (-28.2477, -13.4949)
  line L1725 (-28.2477, -13.4949) -> (-28.2532, -13.5043)
  line L1726 (-28.2532, -13.5043) -> (-28.2563, -13.5067)
  line L1727 (-28.2563, -13.5067) -> (-28.2585, -13.5098)
  line L1728 (-28.2585, -13.5098) -> (-28.2678, -13.5155)
  line L1729 (-28.2678, -13.5155) -> (-28.2764, -13.5221)
  line L1730 (-28.2764, -13.5221) -> (-28.2802, -13.5231)
  line L1731 (-28.2802, -13.5231) -> (-28.2834, -13.5251)
  line L1732 (-28.2834, -13.5251) -> (-28.2942, -13.5269)
  line L1733 (-28.2942, -13.5269) -> (-28.3047, -13.5297)
  line L1734 (-28.3047, -13.5297) -> (-28.3085, -13.5292)
  line L1735 (-28.3085, -13.5292) -> (-28.3123, -13.5298)
  line L1736 (-28.3123, -13.5298) -> (-28.3229, -13.5272)
  line L1737 (-28.3229, -13.5272) -> (-28.3337, -13.5258)
  line L1738 (-28.3337, -13.5258) -> (-28.337, -13.5239)
  line L1739 (-28.337, -13.5239) -> (-28.3408, -13.523)
  line L1740 (-28.3408, -13.523) -> (-28.3496, -13.5166)
  line L1741 (-28.3496, -13.5166) -> (-28.359, -13.5111)
  line L1742 (-28.359, -13.5111) -> (-28.3614, -13.5081)
  line L1743 (-28.3614, -13.5081) -> (-28.3645, -13.5058)
  line L1744 (-28.3645, -13.5058) -> (-28.3702, -13.4966)
  line L1745 (-28.3702, -13.4966) -> (-28.3768, -13.4879)
  line L1746 (-28.3768, -13.4879) -> (-28.3789, -13.4825)
  line L1747 (-28.3789, -13.4825) -> (-28.3798, -13.4809)
  line L1748 (-28.3798, -13.4809) -> (-28.3801, -13.4791)
  line L1749 (-28.3801, -13.4791) -> (-28.382, -13.4741)
  line L1750 (-28.382, -13.4741) -> (-28.5, -13.0316)
  line L1751 (-28.5, -13.0316) -> (-28.618, -13.4741)
  line L1752 (-28.618, -13.4741) -> (-28.6199, -13.4791)
  line L1753 (-28.6199, -13.4791) -> (-28.6202, -13.4809)
  line L1754 (-28.6202, -13.4809) -> (-28.6211, -13.4825)
  line L1755 (-28.6211, -13.4825) -> (-28.6232, -13.4879)
  line L1756 (-28.6232, -13.4879) -> (-28.6298, -13.4966)
  line L1757 (-28.6298, -13.4966) -> (-28.6355, -13.5058)
  line L1758 (-28.6355, -13.5058) -> (-28.6386, -13.5081)
  line L1759 (-28.6386, -13.5081) -> (-28.641, -13.5111)
  line L1760 (-28.641, -13.5111) -> (-28.6504, -13.5166)
  line L1761 (-28.6504, -13.5166) -> (-28.6592, -13.523)
  line L1762 (-28.6592, -13.523) -> (-28.663, -13.5239)
  line L1763 (-28.663, -13.5239) -> (-28.6663, -13.5258)
  line L1764 (-28.6663, -13.5258) -> (-28.6771, -13.5272)
  line L1765 (-28.6771, -13.5272) -> (-28.6877, -13.5298)
  line L1766 (-28.6877, -13.5298) -> (-28.6915, -13.5292)
  line L1767 (-28.6915, -13.5292) -> (-28.6953, -13.5297)
  line L1768 (-28.6953, -13.5297) -> (-28.7058, -13.5269)
  line L1769 (-28.7058, -13.5269) -> (-28.7166, -13.5251)
  line L1770 (-28.7166, -13.5251) -> (-28.7198, -13.5231)
  line L1771 (-28.7198, -13.5231) -> (-28.7236, -13.5221)
  line L1772 (-28.7236, -13.5221) -> (-28.7322, -13.5155)
  line L1773 (-28.7322, -13.5155) -> (-28.7415, -13.5098)
  line L1774 (-28.7415, -13.5098) -> (-28.7437, -13.5067)
  line L1775 (-28.7437, -13.5067) -> (-28.7468, -13.5043)
  line L1776 (-28.7468, -13.5043) -> (-28.7523, -13.4949)
  line L1777 (-28.7523, -13.4949) -> (-28.7586, -13.4861)
  line L1778 (-28.7586, -13.4861) -> (-28.7605, -13.4806)
  line L1779 (-28.7605, -13.4806) -> (-28.7615, -13.479)
  line L1780 (-28.7615, -13.479) -> (-28.7617, -13.4772)
  line L1781 (-28.7617, -13.4772) -> (-28.7634, -13.4722)
  line L1782 (-28.7634, -13.4722) -> (-29.0015, -12.4722)